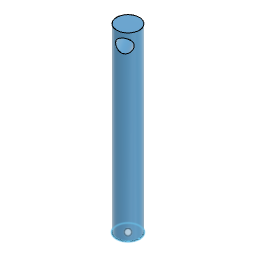
Long Pilon (Autodesk Fusion 360 design; units mm, degrees)
Autodesk Fusion 360 part; units mm, degrees
sketch "sketch 681" plane through (0, 0, 0) normal (0, 0, -1) x (1, 0, 0)
  circle A0 centre (57.5, -105) radius 2.5
  circle A1 centre (57.5, -105) radius 2.5
extrude "Extrude1" add sketch "sketch 681" against normal blind 10
extrude "Extrude2" add 1 faces at (59.187, 104.7086, 10) along direction (0, 0, 1) blind 5
extrude "Extrude3" add 1 faces at (59.187, 104.7086, 15) along direction (0, 0, 1) blind 5
extrude "Extrude4" add 1 faces at (59.187, 104.7086, 20) along direction (0, 0, 1) blind 10
extrude "Extrude5" add 1 faces at (59.187, 104.7086, 30) along direction (0, 0, 1) blind 5
extrude "Extrude6" add 1 faces at (59.187, 104.7086, 35) along direction (0, 0, 1) blind 7
hole "Hole1" at (60, 105, 39.3207) direction (-1, 0, 0) diameter 3 depth 10 tip angle 118
extrude "Extrude7" cut 1 faces at (59.187, 104.7086, 42) along direction (0, 0, -1) blind 7
extrude "Extrude8" add 1 faces at (59.187, 104.7086, 35) along direction (0, 0, 1) blind 5
hole "Hole2" at (-2.6114, 197.4213, 37.4453) direction (0.544639, -0.838671, 0) diameter 3 depth 116 tip angle 118
